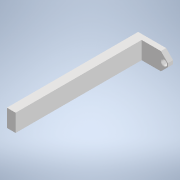
# Autodesk Inventor part: rotator_squarer
Saved by Autodesk Inventor 2022 (Build 260153000, 153)
## iProperties
Created: 2021-07-13
Part Number: rotator_squarer
Material: Generic
Document SubType Name: Modeling
Designer: dsdan
Density: 1 g/cm^3
Appearance: Default
Author: dsdan
Autodesk Inventor part; units mm, degrees
ref_plane "YZ Plane" through (0, 0, 0) normal (1, 0, 0) x (0, 1, 0)
ref_plane "XZ Plane" through (0, 0, 0) normal (0, 1, 0) x (-1, 0, 0)
ref_plane "XY Plane" through (0, 0, 0) normal (0, 0, 1) x (1, 0, 0)
sketch "Sketch1" plane through (0, 0, 0) normal (0, 1, 0) x (-1, 0, 0)
  line L0 (0, 0) -> (10, 0)
  line L1 (10, 0) -> (10, 150)
  line L2 (10, 150) -> (0, 150)
  line L3 (0, 150) -> (0, 0)
  line L4 (0, 6) -> (-34, 6)
  line L5 (-34, 6) -> (-34, 0)
  line L6 (-34, 0) -> (0, 0)
  line L7 (0, 0) -> (0, 6)
  dimension "d0" = 10
  dimension "d1" = 150
  dimension "d2" = 34
  dimension "d3" = 6
  constraints: 16 end point, 4 parallel, 2 horizontal, 2 perpendicular, 2 point on line
  measures "d0" distance between parallel lines of L3 L1
  measures "d1" distance between parallel lines of L2 L0
  measures "d2" distance of L4.start L4.end
  measures "d3" distance between parallel lines of L6 L4
extrude "Extrusion1" add sketch "Sketch1" along normal blind 20
sketch "Sketch2" plane through (0, 0, 6) normal (0, 0, 1) x (1, 0, 0)
  circle A0 centre (25.543, 10) radius 3.1
  line L0 (34, 0) -> (34, 20) projected
  point P0 (0, 0)
  point P1 (34, 10)
  dimension "d6" = 6.2
  dimension "d9" = 8.457
  constraints: 1 centre point, 1 horizontal alignment, 1 midpoint
  measures "d6" diameter of A0
  measures "d9" distance from line of L0 A0.centre
extrude "Extrusion2" cut sketch "Sketch2" against normal through all
chamfer "Chamfer2" distance 1 angle 45 1 edges at (22.443, 10, 6)
sketch "Sketch3" plane through (0, 0, 6) normal (0, 0, 1) x (1, 0, 0)
  line L0 (34, 0) -> (34, 20) projected
  line L1 (34, 5) -> (13, 0)
  line L2 (34, 0) -> (-10, 0) projected
  line L3 (34, 15) -> (13, 20)
  line L4 (0, 20) -> (34, 20) projected
  line L5 (34, 0) -> (34, 20) projected
  circle A0 centre (25.543, 10) radius 3.1 projected
  point P0 (0, 0)
  point P1 (34, 15)
  dimension "d16" = 10
  dimension "d17" = 5
  dimension "d18" = 21
  constraints: 4 end point, 4 point on line, 1 vertical alignment
  measures "d16" distance of L3.start L1.start
  measures "d17" vertical distance of A0.centre L3.start
  measures "d18" horizontal distance of L3.start L3.end
extrude "Extrusion3" cut sketch "Sketch3" against normal through all contours L2 L1 L0 | L3 L4 L0
fillet "Fillet1" radius 4 4 edges at (34, 5, 3) (34, 15, 3) (13, 20, 3) (13, 0, 3)
chamfer "Chamfer3" distance 15 angle 45 1 edges at (0, 10, 6)
equation "\"d17\" = 0.5 * d16"
body "Solid1"
